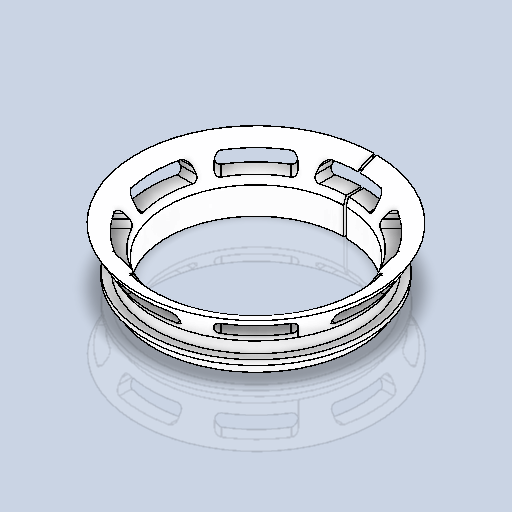
# Autodesk Inventor part: Glove_ring
Saved by Autodesk Inventor 2026.1 (Build 301233000, 233)
## iProperties
Created: 2025-08-29
Part Number: Glove_ring
Material: Aluminum 6061
Document SubType Name: Modeling
Designer: baseb
Density: 2.7 g/cm^3
Appearance: Aluminum - Flat
Author: baseb
Autodesk Inventor part; units mm, degrees
ref_plane "YZ Plane" through (0, 0, 0) normal (1, 0, 0) x (0, 1, 0)
ref_plane "XZ Plane" through (0, 0, 0) normal (0, 1, 0) x (-1, 0, 0)
sketch "Sketch2" plane through (0, 0, 0) normal (1, 0, 0) x (0, 1, 0)
  line L0 (0, 0) -> (0, -17.145)
  line L1 (0, -17.145) -> (34.925, -17.145)
  line L2 (34.925, -17.145) -> (34.925, 0)
  line L3 (34.925, 0) -> (0, 0)
  line L4 (34.925, 0) -> (73.025, 21.997)
  line L5 (34.925, 0) -> (78.9191, 0) construction
  arc A0 (34.925, -17.145) -> (73.025, 21.997) centre (24.06, 31.5447) ccw
  line L6 (0, -17.145) -> (0, -131.445) construction
  line L7 (0, -131.445) -> (102.4655, -131.445)
  line L8 (20.6375, 0) -> (20.6375, 9.525)
  line L9 (20.6375, 9.525) -> (14.2875, 9.525)
  line L10 (14.2875, 9.525) -> (14.2875, 0)
  point P0 (17.4625, 0)
  dimension "d2" = 34.925
  dimension "d3" = 17.145
  dimension "d6" = 30
  dimension "d7" = 114.3
  dimension "d9" = 6.35
  dimension "d10" = 9.525
  constraints: 22 end point, 3 perpendicular, 2 horizontal, 2 point on circle, 2 point on line, 2 vertical, 1 centre point, 1 equal length, 1 midpoint, 1 parallel
  measures "d2" distance of L0.end L1.end
  measures "d3" distance of L1.end L2.end
  measures "d6" angle of L5 L4
  measures "d7" distance of L0.end L6.end
  measures "d9" distance of L8.end L9.end
  measures "d10" distance between parallel lines of L3 L9
revolve "Revolution1" add sketch "Sketch2" angle 360 about axis through (0, 0, -131.445) along (0, 1, 0)
sketch "Sketch4" plane through (0, 0, -131.445) normal (0, -1, 0) x (1, 0, 0)
  line L0 (1.5875, -60.2816) -> (-1.5875, -60.2816)
  line L1 (-1.5875, -60.2816) -> (-1.5875, -168.3184)
  line L2 (-1.5875, -168.3184) -> (1.5875, -168.3184)
  line L3 (1.5875, -168.3184) -> (1.5875, -60.2816)
  circle A0 centre (0, 0) radius 114.3 projected
  line L4 (1.5875, -60.2816) -> (-1.5875, -168.3184) construction
  line L5 (-1.5875, -60.2816) -> (1.5875, -168.3184) construction
  point P0 (0, 131.445)
  point P1 (0, -114.3)
  dimension "d17" = 3.175
  constraints: 12 end point, 2 midpoint, 2 parallel, 1 horizontal, 1 perpendicular, 1 vertical alignment, 1 other
  measures "d17" distance of L1.end L2.end
extrude "Extrusion2" cut sketch "Sketch4" against normal through all contours L3 A0 L1 L0 | L3 L2 L1 A0 picked at (0.1764, -78.2873)
sketch "Sketch5" plane through (0, 0, -131.445) normal (0, -1, 0) x (1, 0, 0)
  arc A0 (1.5875, -131.4354) -> (-1.5875, -131.4354) centre (0, 0) ccw projected
  line L0 (32.0945, -127.4666) -> (1.5875, -140.9611)
  line L1 (1.5875, -140.9611) -> (21.7532, -140.9611)
  line L2 (21.7532, -140.9611) -> (32.0945, -127.4666)
  line L3 (0, -127.4666) -> (0, -140.9122)
  line L4 (-32.0945, -127.4666) -> (-1.5875, -140.9611)
  line L5 (-1.5875, -140.9611) -> (-21.7532, -140.9611)
  line L6 (-21.7532, -140.9611) -> (-32.0945, -127.4666)
  arc A1 (-32.0945, -127.4666) -> (32.0945, -127.4666) centre (0, 0) ccw
  line L7 (1.5875, -140.9611) -> (1.5875, -131.4354)
  line L8 (-1.5875, -140.9611) -> (-1.5875, -131.4354) projected
  line L9 (-1.5875, -140.9611) -> (-1.5875, -131.4354)
  point P0 (0, 131.445)
  point P1 (-32.0945, -127.4666)
  constraints: 18 end point, 3 point on circle, 3 symmetric about line, 1 centre point, 1 collinear, 1 horizontal, 1 parallel, 1 vertical
extrude "Extrusion3" add sketch "Sketch5" against normal blind 34.925 contours A0 L0 L7 | L2 L1 L0 | A0 L8 L4 | L4 L5 L6
sketch "Sketch6" plane through (0, 14.2875, -131.445) normal (0, -1, 0) x (1, 0, 0)
  arc A0 (-32.0945, -127.4666) -> (-1.5875, -131.4354) centre (0, 0) ccw projected
  line L0 (0, 0) -> (32.0945, -127.4666) construction
  line L1 (32.0945, -127.4666) -> (34.4202, -136.7033)
  arc A1 (23.2222, -139.0441) -> (-23.2222, -139.0441) centre (0, 0) ccw projected
  line L2 (23.2222, -139.0441) -> (32.0945, -127.4666) projected
  line L3 (32.0945, -127.4666) -> (23.2222, -139.0441)
  line L4 (32.0945, -127.4666) -> (60.2091, -127.4653)
  arc A2 (34.4202, -136.7033) -> (60.2091, -127.4653) centre (-0.0009, 0.0024) ccw
  line L5 (-0.0009, 0.0024) -> (-32.0945, -127.4666) construction
  line L6 (-34.4201, -136.7033) -> (-32.0945, -127.4666)
  line L7 (-32.0945, -127.4666) -> (-23.2222, -139.0441)
  line L8 (-21.7532, -140.9611) -> (-32.0945, -127.4666) projected
  line L9 (-32.0945, -127.4666) -> (-60.2085, -127.4656)
  arc A3 (-23.2222, -139.0441) -> (-34.4201, -136.7033) centre (0, 0) ccw
  arc A4 (-34.4201, -136.7033) -> (-60.2085, -127.4656) centre (0, 0) ccw
  point P0 (0, 131.445)
  point P1 (-30.3188, -129.7837)
  dimension "d24" = 75.87
  dimension "d25" = 51.597
  dimension "d26" = 51.596
  dimension "d27" = 75.87
  constraints: 16 end point, 11 point on circle, 3 centre point, 3 collinear, 2 point on line, 1 concentric
  measures "d24" angle of L4 L1
  measures "d25" angle of L2 L1
  measures "d26" angle of L6 L7
  measures "d27" angle of L9 L6
extrude "Extrusion4" cut sketch "Sketch6" against normal up to surface (6.35 mm away) contours L4 A1 L1 | L1 A1 L2 | A1 L6 L7 | L9 L6 A1
ref_plane "Work Plane1" through (32.0945, 17.4625, -258.9116) normal (1, 0, 0) x (0, 0, -1)
sketch "Sketch7" plane through (32.0945, 17.4625, -258.9116) normal (1, 0, 0) x (0, 0, -1)
  circle A0 centre (6.7472, 0) radius 3.175
  line L0 (0, -17.4625) -> (13.4945, -17.4625) projected
  line L1 (6.7472, -17.4625) -> (6.7472, 0) construction
  point P0 (-258.9116, -17.4625)
  constraints: 2 end point, 1 centre point, 1 midpoint, 1 vertical
extrude "Extrusion5" cut sketch "Sketch7" against normal through all
sketch "Sketch3" plane through (0, 0, 0) normal (0, 0, 1) x (1, 0, 0)
  line L0 (-31.75, 63.5) -> (31.75, 63.5)
  line L1 (38.1, 57.15) -> (38.1, 50.8)
  line L2 (31.75, 44.45) -> (-31.75, 44.45)
  line L3 (-38.1, 50.8) -> (-38.1, 57.15)
  line L4 (-38.1, 63.5) -> (38.1, 44.45) construction
  line L5 (38.1, 63.5) -> (-38.1, 44.45) construction
  line L6 (153.442, 73.025) -> (-153.442, 73.025) projected
  line L7 (0, 44.45) -> (0, 63.5)
  arc A0 (-38.1, 50.8) -> (-31.75, 44.45) centre (-31.75, 50.8) ccw
  arc A1 (31.75, 44.45) -> (38.1, 50.8) centre (31.75, 50.8) ccw
  arc A2 (38.1, 57.15) -> (31.75, 63.5) centre (31.75, 57.15) ccw
  arc A3 (-31.75, 63.5) -> (-38.1, 57.15) centre (-31.75, 57.15) ccw
  point P0 (0, 0)
  point P1 (0, 53.975)
  dimension "d11" = 19.05
  dimension "d12" = 9.525
  dimension "d13" = 76.2
  dimension "d14" = 0
  dimension "d36" = 6.35
  constraints: 14 end point, 8 point on circle, 8 point on line, 8 tangent, 4 centre point, 4 midpoint, 3 equal radius, 2 parallel, 1 horizontal, 1 perpendicular
  measures "d11" distance of L5.start L4.end
  measures "d12" distance between parallel lines of L6 L0
  measures "d13" distance of L4.end L5.end
  measures "d14" distance from line of point (0, 0) L7
  measures "d36" radius of A0
extrude "Extrusion1" cut sketch "Sketch3" along normal through all both and the other way through all
pattern_circular "Circular Pattern1" count 8 over 360 about axis through (0, 17.4625, -131.445) along (0, 1, 0) of "Extrusion1"
equation "\"d27\" = d24"
equation "\"d13\" = 4 * d11"
body "Solid1"
